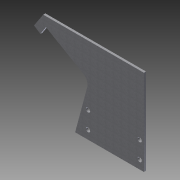
# Autodesk Inventor part: plate_metal_hook
Saved by Autodesk Inventor 2011 (Build 150239000, 239)
## iProperties
Created: 2013-01-17
Part Number: plate_metal_hook
Document SubType Name: Modeling
Designer: Christopher
Density: 1 g/cm^3
Author: Christopher
Autodesk Inventor part; units mm, degrees
ref_plane "YZ Plane" through (0, 0, 0) normal (1, 0, 0) x (0, 1, 0)
ref_plane "XZ Plane" through (0, 0, 0) normal (0, 1, 0) x (-1, 0, 0)
ref_plane "XY Plane" through (0, 0, 0) normal (0, 0, 1) x (1, 0, 0)
sketch "Sketch1" plane through (0, 0, 0) normal (0, 0, 1) x (1, 0, 0)
  line L0 (94.9487, -77.075) -> (183.8487, -77.075)
  line L1 (94.9487, -77.075) -> (82.2487, -77.075)
  line L2 (82.2487, -77.075) -> (102.6664, -0.875)
  line L3 (183.8487, 49.925) -> (183.8487, -77.075)
  line L4 (183.8487, 49.925) -> (35.0711, 49.925)
  line L5 (102.6664, -0.875) -> (39.1664, 35.7867)
  line L6 (39.1664, 35.7867) -> (30.7882, 23.0867)
  line L7 (30.7882, 23.0867) -> (21.436, 29.2563)
  line L8 (21.436, 29.2563) -> (35.0711, 49.925)
  point P0 (0, 0)
  point P1 (177.5476, -64.375)
  point P2 (177.5476, -38.975)
  point P3 (101.3476, -38.975)
  point P4 (101.3476, -64.375)
  dimension "d3" = 88.9
  dimension "d9" = 76.2
  dimension "d10" = 25.4
  dimension "d11" = 12.7
  dimension "d22" = 12.7
  dimension "d24" = 76.2
  dimension "d29" = 127
  dimension "d32" = 75
  dimension "d33" = 105
  dimension "d34" = 12.7
  dimension "d35" = 63.5
  constraints: 18 end point, 5 perpendicular, 2 horizontal alignment, 2 vertical alignment, 1 horizontal
  measures "d3" distance of L0.start L0.end
  measures "d9" distance of point (177.548, -64.375) point (101.348, -64.375)
  measures "d10" distance of point (101.348, -64.375) point (101.348, -38.975)
  measures "d11" distance from line of L0 point (101.348, -64.375)
  measures "d22" distance of L0.start L1.end
  measures "d24" vertical distance of L1.end L2.end
  measures "d29" distance of L3.start L0.end
  measures "d32" angle of L0 L2
  measures "d33" angle of L2 L5
  measures "d34" vertical distance of L5.end L6.end
  measures "d35" horizontal distance of L2.end L5.end
extrude "Extrusion1" add sketch "Sketch1" against normal blind 3.175
hole "Hole1" at (177.5476, -64.375, 0) at (177.5476, -38.975, 0) at (101.3476, -38.975, 0) at (101.3476, -64.375, 0) direction (0, 0, -1) diameter 6.35 depth 25.4 tip angle 118
fillet "Fillet1" radius 12.7 1 edges at (102.6664, -0.875, -1.5875)
body "Solid1"
